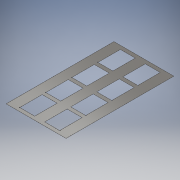
# Autodesk Inventor part: Assembly Stencil
Saved by Autodesk Inventor 2019.4 (Build 234330000, 330)
## iProperties
Created: 2021-01-11
Part Number: Assembly Stencil
Material: Stainless Steel
Document SubType Name: Modeling
Designer: caleb
Density: 8 g/cm^3
Appearance: Semi-Polished
Author: caleb
Autodesk Inventor part; units mm, degrees
ref_plane "YZ Plane" through (0, 0, 0) normal (1, 0, 0) x (0, 1, 0)
ref_plane "XZ Plane" through (0, 0, 0) normal (0, 1, 0) x (-1, 0, 0)
ref_plane "XY Plane" through (0, 0, 0) normal (0, 0, 1) x (1, 0, 0)
sketch "Sketch1" plane through (0, 0, 0) normal (0, 1, 0) x (-1, 0, 0)
  line L0 (-60, 108) -> (60, 108)
  line L1 (60, 108) -> (60, -108)
  line L2 (60, -108) -> (-60, -108)
  line L3 (-60, -108) -> (-60, 108)
  line L4 (-60, 108) -> (60, -108) construction
  line L5 (60, 108) -> (-60, -108) construction
  point P0 (0, 0)
  dimension "d0" = 216
  dimension "d1" = 120
  constraints: 12 end point, 2 midpoint, 2 parallel, 1 horizontal, 1 perpendicular
  measures "d0" distance of L0.end L1.end
  measures "d1" distance of L0.start L0.end
extrude "Extrusion1" add sketch "Sketch1" along normal blind 0.1
sketch "Sketch2" plane through (0, 0.1, 0) normal (0, 1, 0) x (1, 0, 0)
  line L0 (-39.8, -100.8) -> (-10.2, -100.8)
  line L1 (-10, -100.6) -> (-10, -56)
  line L2 (-10.2, -55.8) -> (-39.8, -55.8)
  line L3 (-40, -56) -> (-40, -100.6)
  line L4 (-60, -108) -> (60, -108) projected
  line L5 (-60, 108) -> (-60, -108) projected
  circle A0 centre (-40, -100.8) radius 1
  arc A1 (-39.8, -55.8) -> (-40, -56) centre (-39.8, -56) ccw
  arc A2 (-10, -56) -> (-10.2, -55.8) centre (-10.2, -56) ccw
  arc A3 (-10.2, -100.8) -> (-10, -100.6) centre (-10.2, -100.6) ccw
  arc A4 (-40, -100.6) -> (-39.8, -100.8) centre (-39.8, -100.6) ccw
  arc A5 (-10.2, -48.6) -> (-10, -48.4) centre (-10.2, -48.4) ccw
  line L6 (-10, -48.4) -> (-10, -3.8)
  arc A6 (-10, -3.8) -> (-10.2, -3.6) centre (-10.2, -3.8) ccw
  line L7 (-39.8, -48.6) -> (-10.2, -48.6)
  arc A7 (-40, -48.4) -> (-39.8, -48.6) centre (-39.8, -48.4) ccw
  line L8 (-10.2, -3.6) -> (-39.8, -3.6)
  arc A8 (-39.8, -3.6) -> (-40, -3.8) centre (-39.8, -3.8) ccw
  line L9 (-40, -3.8) -> (-40, -48.4)
  arc A9 (-10.2, 3.6) -> (-10, 3.8) centre (-10.2, 3.8) ccw
  line L10 (-10, 3.8) -> (-10, 48.4)
  arc A10 (-10, 48.4) -> (-10.2, 48.6) centre (-10.2, 48.4) ccw
  line L11 (-39.8, 3.6) -> (-10.2, 3.6)
  arc A11 (-40, 3.8) -> (-39.8, 3.6) centre (-39.8, 3.8) ccw
  line L12 (-10.2, 48.6) -> (-39.8, 48.6)
  arc A12 (-39.8, 48.6) -> (-40, 48.4) centre (-39.8, 48.4) ccw
  line L13 (-40, 48.4) -> (-40, 3.8)
  arc A13 (-10.2, 55.8) -> (-10, 56) centre (-10.2, 56) ccw
  line L14 (-10, 56) -> (-10, 100.6)
  arc A14 (-10, 100.6) -> (-10.2, 100.8) centre (-10.2, 100.6) ccw
  line L15 (-39.8, 55.8) -> (-10.2, 55.8)
  arc A15 (-40, 56) -> (-39.8, 55.8) centre (-39.8, 56) ccw
  line L16 (-10.2, 100.8) -> (-39.8, 100.8)
  arc A16 (-39.8, 100.8) -> (-40, 100.6) centre (-39.8, 100.6) ccw
  line L17 (-40, 100.6) -> (-40, 56)
  arc A17 (39.8, -100.8) -> (40, -100.6) centre (39.8, -100.6) ccw
  line L18 (40, -100.6) -> (40, -56)
  arc A18 (40, -56) -> (39.8, -55.8) centre (39.8, -56) ccw
  line L19 (10.2, -100.8) -> (39.8, -100.8)
  arc A19 (10, -100.6) -> (10.2, -100.8) centre (10.2, -100.6) ccw
  line L20 (39.8, -55.8) -> (10.2, -55.8)
  arc A20 (10.2, -55.8) -> (10, -56) centre (10.2, -56) ccw
  line L21 (10, -56) -> (10, -100.6)
  arc A21 (39.8, -48.6) -> (40, -48.4) centre (39.8, -48.4) ccw
  line L22 (40, -48.4) -> (40, -3.8)
  arc A22 (40, -3.8) -> (39.8, -3.6) centre (39.8, -3.8) ccw
  line L23 (10.2, -48.6) -> (39.8, -48.6)
  arc A23 (10, -48.4) -> (10.2, -48.6) centre (10.2, -48.4) ccw
  line L24 (39.8, -3.6) -> (10.2, -3.6)
  arc A24 (10.2, -3.6) -> (10, -3.8) centre (10.2, -3.8) ccw
  line L25 (10, -3.8) -> (10, -48.4)
  arc A25 (39.8, 3.6) -> (40, 3.8) centre (39.8, 3.8) ccw
  line L26 (40, 3.8) -> (40, 48.4)
  arc A26 (40, 48.4) -> (39.8, 48.6) centre (39.8, 48.4) ccw
  line L27 (10.2, 3.6) -> (39.8, 3.6)
  arc A27 (10, 3.8) -> (10.2, 3.6) centre (10.2, 3.8) ccw
  line L28 (39.8, 48.6) -> (10.2, 48.6)
  arc A28 (10.2, 48.6) -> (10, 48.4) centre (10.2, 48.4) ccw
  line L29 (10, 48.4) -> (10, 3.8)
  arc A29 (39.8, 55.8) -> (40, 56) centre (39.8, 56) ccw
  line L30 (40, 56) -> (40, 100.6)
  arc A30 (40, 100.6) -> (39.8, 100.8) centre (39.8, 100.6) ccw
  line L31 (10.2, 55.8) -> (39.8, 55.8)
  arc A31 (10, 56) -> (10.2, 55.8) centre (10.2, 56) ccw
  line L32 (39.8, 100.8) -> (10.2, 100.8)
  arc A32 (10.2, 100.8) -> (10, 100.6) centre (10.2, 100.6) ccw
  line L33 (10, 100.6) -> (10, 56)
  circle A33 centre (-40, -48.6) radius 1
  circle A34 centre (-40, 3.6) radius 1
  circle A35 centre (-40, 55.8) radius 1
  circle A36 centre (40, -100.8) radius 1
  circle A37 centre (40, -48.6) radius 1
  circle A38 centre (40, 3.6) radius 1
  circle A39 centre (40, 55.8) radius 1
  point P0 (0, 0)
  point P1 (-10, -100.8)
  point P2 (-40, -55.8)
  point P3 (-10, -48.6)
  point P4 (-40, -3.6)
  point P5 (-10, 3.6)
  point P6 (-40, 48.6)
  point P7 (-10, 55.8)
  point P8 (-40, 100.8)
  point P9 (40, -100.8)
  point P10 (10, -100.8)
  point P11 (10, -100.8)
  point P12 (10, -55.8)
  point P13 (40, -48.6)
  point P14 (10, -48.6)
  point P15 (10, -48.6)
  point P16 (10, -3.6)
  point P17 (40, 3.6)
  point P18 (10, 3.6)
  point P19 (10, 3.6)
  point P20 (10, 48.6)
  point P21 (40, 55.8)
  point P22 (10, 55.8)
  point P23 (10, 55.8)
  point P24 (10, 100.8)
  dimension "d4" = 30
  dimension "d5" = 45
  dimension "d6" = 7.2
  dimension "d7" = 20
  dimension "d8" = 2
  dimension "d9" = 0.2
  dimension "d20" = 0.2
  dimension "d23" = 52.2
  dimension "d26" = 50
  dimension "d31" = 52.2
  dimension "d34" = 80
  constraints: 64 end point, 64 point on circle, 48 point on line, 40 centre point, 8 coincident, 8 tangent, 3 horizontal, 2 equal radius, 2 parallel, 2 vertical, 1 perpendicular, 182 other
  measures "d4" distance of point (-40, -100.8) point (-10, -100.8)
  measures "d5" distance of point (-40, -55.8) point (-40, -100.8)
  measures "d6" distance between parallel lines of L4 L0
  measures "d7" distance between parallel lines of L5 L3
  measures "d8" diameter of A0
  measures "d9" radius of A1
  measures "d20" radius of A4
  measures "d23" distance of point (-10, -100.8) point (-10, -48.6)
  measures "d26" distance of point (-10, -100.8) point (40, -100.8)
  measures "d31" distance of A0.centre A33.centre
  measures "d34" distance of A0.centre A36.centre
extrude "Extrusion2" cut sketch "Sketch2" against normal through all
body "Solid1"
